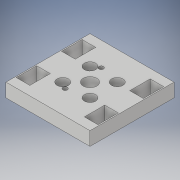
# Autodesk Inventor part: thumper-base-v3
Saved by Autodesk Inventor 2017 (Build 210142000, 142)
## iProperties
Created: 2017-02-22
Part Number: thumper-base-v3
Material: Generic
Document SubType Name: Modeling
Designer: John
Density: 1 g/cm^3
Appearance: Default
Author: John
Autodesk Inventor part; units mm, degrees
ref_plane "YZ Plane" through (0, 0, 0) normal (1, 0, 0) x (0, 1, 0)
ref_plane "XZ Plane" through (0, 0, 0) normal (0, 1, 0) x (-1, 0, 0)
ref_plane "XY Plane" through (0, 0, 0) normal (0, 0, 1) x (1, 0, 0)
sketch "Sketch2" plane through (0, 0, 0) normal (0, 1, 0) x (-1, 0, 0)
  line L0 (-18.5, 18.5) -> (18.5, 18.5)
  line L1 (18.5, 18.5) -> (18.5, -18.5)
  line L2 (18.5, -18.5) -> (-18.5, -18.5)
  line L3 (-18.5, -18.5) -> (-18.5, 18.5)
  line L4 (-18.5, 18.5) -> (18.5, -18.5) construction
  line L5 (18.5, 18.5) -> (-18.5, -18.5) construction
  line L6 (12, -14.5) -> (18, -14.5)
  line L7 (18, -14.5) -> (18, -5.5)
  line L8 (18, -5.5) -> (12, -5.5)
  line L9 (12, -5.5) -> (12, -14.5)
  line L10 (12, -14.5) -> (18, -5.5) construction
  line L11 (18, -14.5) -> (12, -5.5) construction
  line L12 (0, 18.5) -> (0, -18.5) construction
  line L13 (18.5, 0) -> (-18.5, 0) construction
  circle A0 centre (0, 0) radius 3
  circle A1 centre (6, -6) radius 2.5
  circle A2 centre (-6, 6) radius 2.5
  circle A3 centre (3, -7.953) radius 1
  line L14 (12, 14.5) -> (18, 14.5)
  line L15 (18, 14.5) -> (18, 5.5)
  line L16 (18, 5.5) -> (12, 5.5)
  line L17 (12, 5.5) -> (12, 14.5)
  line L18 (12, 14.5) -> (18, 5.5) construction
  line L19 (18, 14.5) -> (12, 5.5) construction
  line L20 (-12, -14.5) -> (-18, -14.5)
  line L21 (-18, -14.5) -> (-18, -5.5)
  line L22 (-18, -5.5) -> (-12, -5.5)
  line L23 (-12, -5.5) -> (-12, -14.5)
  line L24 (-12, -14.5) -> (-18, -5.5) construction
  line L25 (-18, -14.5) -> (-12, -5.5) construction
  line L26 (-12, 5.5) -> (-12, 14.5)
  line L27 (-12, 14.5) -> (-18, 14.5)
  line L28 (-18, 14.5) -> (-18, 5.5)
  line L29 (-12, 14.5) -> (-18, 5.5) construction
  line L30 (-18, 14.5) -> (-12, 5.5) construction
  line L31 (-18, 5.5) -> (-12, 5.5)
  circle A4 centre (6, 6) radius 2.5
  circle A5 centre (-6, -6) radius 2.5
  circle A6 centre (3, 7.953) radius 1
  point P0 (15, -10)
  point P1 (15, 10)
  point P2 (-15, -10)
  point P3 (-15, 10)
  dimension "d0" = 37
  dimension "d1" = 37
  dimension "d3" = 9
  dimension "d5" = 6
  dimension "d8" = 5
  dimension "d10" = 6
  dimension "d11" = 6
  dimension "d23" = 2
  dimension "d27" = 6
  dimension "d30" = 15
  dimension "d32" = 14.5
  dimension "d33" = 9
  dimension "d35" = 8.5
  constraints: 64 end point, 19 symmetric about line, 14 midpoint, 7 centre point, 4 parallel, 2 horizontal, 2 perpendicular, 1 coincident, 4 other
  measures "d0" distance of L1.end L2.end
  measures "d1" distance of L0.end L1.end
  measures "d3" distance of L7.end L6.end
  measures "d5" diameter of A0
  measures "d8" diameter of A1
  measures "d10" horizontal distance of point (0, 0) A1.centre
  measures "d11" horizontal distance of A0.centre A1.centre
  measures "d23" diameter of A3
  measures "d27" distance of L7.end L8.end
  measures "d30" horizontal distance of point (0, 0) point (15, -10)
  measures "d32" distance between parallel lines of L13 L6
  measures "d33" distance from line of L9 A3.centre
  measures "d35" distance of A3.centre point (0, 0)
extrude "Extrusion1" add sketch "Sketch2" along normal blind 6
equation "\"d0\" = d1"
equation "\"d11\" = d10"
body "Solid1"
